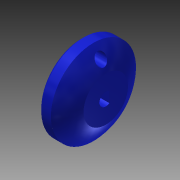
# Autodesk Inventor part: Flexiwheel Hub - Motor Side
Saved by Autodesk Inventor 2014 (Build 180170000, 170)
## iProperties
Created: 2014-02-03
Part Number: Flexiwheel Hub - Motor Side
Material: Generic
Document SubType Name: Modeling
Designer: Spooner
Density: 1 g/cm^3
Appearance: Blue - Wall Paint - Glossy
Author: Spooner
Autodesk Inventor part; units mm, degrees
ref_plane "XZ Plane" through (0, 0, 0) normal (0, 1, 0) x (-1, 0, 0)
ref_plane "XY Plane" through (0, 0, 0) normal (0, 0, 1) x (1, 0, 0)
sketch "Sketch1" plane through (0, 0, 0) normal (0, 0, 1) x (1, 0, 0)
  line L0 (0, 0) -> (-8.052, 0) construction
  line L1 (-6.096, 2.032) -> (5.08, 2.032)
  line L2 (-6.096, 2.032) -> (-6.096, 3.2258)
  line L3 (-6.096, 3.2258) -> (0, 3.2258)
  line L4 (0, 3.2258) -> (0, 6.9215)
  line L5 (0, 6.9215) -> (-3.81, 6.9215)
  line L6 (-3.81, 6.9215) -> (-3.81, 13.5001)
  line L7 (-3.81, 13.5001) -> (0, 13.5001)
  arc A0 (5.08, 2.032) -> (0, 13.5001) centre (-14.9919, 0) ccw
  dimension "d0" = 2.032
  dimension "d1" = 13.5001
  dimension "d2" = 6.096
  dimension "d3" = 3.2258
  dimension "d4" = 3.81
  dimension "d5" = 6.9215
  dimension "d7" = 5.08
  constraints: 16 end point, 5 parallel, 2 perpendicular, 2 point on circle, 2 vertical alignment, 1 centre point, 1 horizontal, 1 point on line
  measures "d0" distance between parallel lines of L0 L1
  measures "d1" distance between parallel lines of L0 L7
  measures "d2" distance from line of L2 L7.end
  measures "d3" distance between parallel lines of L0 L3
  measures "d4" distance from line of L7.end L6
  measures "d5" distance between parallel lines of L0 L5
  measures "d7" horizontal distance of L0.start L1.end
revolve "Revolution1" add sketch "Sketch1" angle 360 about axis through (0, 0, 0) along (-1, 0, 0)
ref_plane "Work Plane3" through (3.9126, 0, 0) normal (1, 0, 0) x (0, 1, 0)
ref_plane "Work Plane2" through (5.1826, 0, 0) normal (1, 0, 0) x (0, 1, 0)
sketch "Sketch2" plane through (3.9126, 0, 0) normal (1, 0, 0) x (0, 1, 0)
  circle A0 centre (0, 0) radius 2.032 projected
  line L0 (-1.6801, -1.143) -> (1.6801, -1.143)
  dimension "d10" = 3.175
  constraints: 2 end point, 2 point on circle, 1 horizontal
extrude "Extrusion1" add sketch "Sketch2" against normal blind 6.604 contours L0 A0 picked at (-0.4517, -1.2667)
sketch "Sketch3" plane through (-2.6914, 0, 0) normal (-1, 0, 0) x (0, 0, 1)
  arc A0 (-1.143, 1.6801) -> (-1.143, -1.6801) centre (0, 0) ccw projected
  line L0 (-1.143, -1.6801) -> (-1.143, 1.6801) projected
  circle A1 centre (0, 0) radius 1.143
  circle A2 centre (0, 0) radius 2.032 projected
  dimension "d13" = 2.286
  constraints: 1 centre point, 1 coincident
  measures "d13" diameter of A1
extrude "Extrusion2" add sketch "Sketch3" along normal up to surface (3.4046 mm away)
sketch "Sketch4" plane through (-3.81, 0, 0) normal (-1, 0, 0) x (0, 0, 1)
  circle A0 centre (0, 10.16) radius 1.7272 projected
extrude "Extrusion3" cut sketch "Sketch4" against normal through all
chamfer "Chamfer1" distance 0.762 angle 45 4 edges at (-3.81, -13.5001, 0) (-3.81, -6.9215, 0) (-6.096, -3.2258, 0) (-6.096, 0, -1.143)
sketch "Sketch5" plane through (3.9126, 0, 0) normal (1, 0, 0) x (0, 1, 0)
  circle A0 centre (0, 0) radius 22.931
  constraints: 1 centre point, 1 coincident
extrude "Extrusion4" cut sketch "Sketch5" along normal blind 25.4
body "Solid1"
